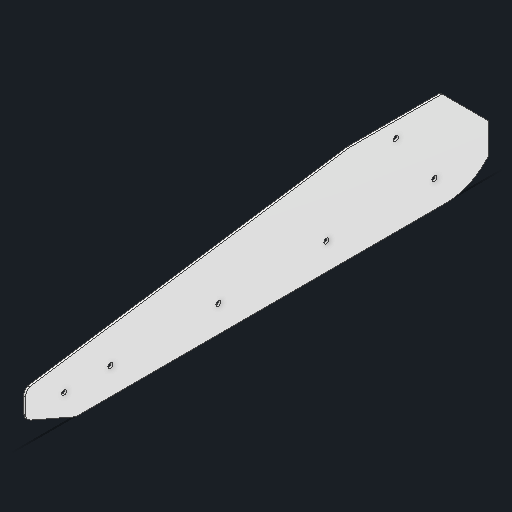
# Autodesk Inventor part: Skirt
Saved by Autodesk Inventor 2025.1 (Build 291241000, 241)
## iProperties
Created: 2024-10-17
Part Number: Skirt
Material: Acetal Resin, White
Document SubType Name: Sheet Metal
Designer: averey
Density: 1.425 g/cm^3
Appearance: Smooth - White
Mass: 37.0306 g
Surface Area: 482.458 cm^2
Volume: 37.0306 cm^3
Flat Pattern Width: 7.9375 cm
Flat Pattern Length: 38.1 cm
Flat Pattern Area: 302.419 cm^2
Sheet Metal Rule: Default_mm
Sheet Metal Width: 3.125 in
Sheet Metal Length: 15.000 in
Sheet Metal Area: 46.875 in^2
d0: 0.500 in
d1: 12.000 in
d2: 0.625 in
d3: 1.000 in
d4: 0.125 in
d8: 0.165 in
Author: averey
Autodesk Inventor part; units mm, degrees
ref_plane "YZ Plane" through (0, 0, 0) normal (1, 0, 0) x (0, 1, 0)
ref_plane "XZ Plane" through (0, 0, 0) normal (0, 1, 0) x (-1, 0, 0)
ref_plane "XY Plane" through (0, 0, 0) normal (0, 0, 1) x (1, 0, 0)
sketch "main" plane through (0, 0, 0) normal (0, 0, 1) x (1, 0, 0)
  circle A0 centre (-12.3674, 169.8166) radius 2.0955
  circle A1 centre (-12.3674, 131.7166) radius 2.0955
  circle A2 centre (-12.3674, 42.8166) radius 2.0955
  circle A3 centre (-12.3674, -46.0834) radius 2.0955
  circle A4 centre (-12.3674, -134.9834) radius 2.0955
  arc A5 (6.5152, 193.7683) -> (0.3326, 201.5666) centre (0.3326, 195.2166) ccw
  line L0 (-34.5924, 159.4847) -> (-34.5924, -144.653)
  line L1 (5.8319, 198.3916) -> (44.7826, -65.1334)
  arc A6 (-34.3276, 160.7541) -> (-34.5924, 159.4847) centre (-31.4174, 159.4847) ccw
  line L2 (-34.3276, 160.7541) -> (-18.1878, 197.7554)
  line L3 (0.3326, 201.5666) -> (-12.3674, 201.5666)
  arc A7 (-12.3674, 201.5666) -> (-18.1878, 197.7554) centre (-12.3674, 195.2166) ccw
  line L4 (44.7826, -65.1334) -> (44.7826, -141.3334)
  arc A8 (-34.5924, -144.653) -> (-18.7174, -179.4334) centre (11.4451, -144.653) ccw
  line L5 (6.6826, -179.4334) -> (-18.7174, -179.4334)
  line L6 (44.7826, -141.3334) -> (6.6826, -179.4334)
  circle A9 centre (32.0826, -103.2334) radius 2.0955
  point P0 (-1.329, 35.5886)
  point P1 (-34.5924, 160.147)
  point P2 (38.4326, -84.1834)
  dimension "d0" = 12.7
  dimension "d1" = 304.8
  dimension "d2" = 15.875
  dimension "d3" = 25.4
  dimension "d4" = 3.175
  dimension "d8" = 4.191
  dimension "d9" = 4.191
  dimension "d10" = 4.191
  dimension "d11" = 4.191
  dimension "d12" = 4.191
  dimension "d13" = 4.191
  measures "d0" diameter of A5
  measures "d1" distance of point (-34.592, 160.147) L0.end
  measures "d2" distance from line of L5.end L0
  measures "d3" distance of L6.end L5.end
  measures "d4" radius of A6
  measures "d8" diameter of A9
  measures "d9" diameter of A3
  measures "d10" diameter of A4
  measures "d11" diameter of A2
  measures "d12" diameter of A1
  measures "d13" diameter of A0
sketch "Sketch1" plane through (0, 0, 0) normal (1, 0, 0) x (0, 1, 0)
  circle A0 centre (0, 0) radius 2.0955
  circle A1 centre (0, -38.1) radius 2.0955
  circle A2 centre (0, -127) radius 2.0955
  circle A3 centre (0, -215.9) radius 2.0955
  circle A4 centre (0, -304.8) radius 2.0955
  arc A5 (18.8826, 23.9517) -> (12.7, 31.75) centre (12.7, 25.4) ccw
  line L0 (-22.225, -10.3319) -> (-22.225, -314.4696)
  line L1 (18.1993, 28.575) -> (57.15, -234.95)
  arc A6 (-21.9602, -9.0625) -> (-22.225, -10.3319) centre (-19.05, -10.3319) ccw
  line L2 (-21.9602, -9.0625) -> (-5.8204, 27.9388)
  line L3 (12.7, 31.75) -> (0, 31.75)
  arc A7 (0, 31.75) -> (-5.8204, 27.9388) centre (0, 25.4) ccw
  line L4 (57.15, -234.95) -> (57.15, -311.15)
  arc A8 (-22.225, -314.4696) -> (-6.35, -349.25) centre (23.8125, -314.4696) ccw
  line L5 (19.05, -349.25) -> (-6.35, -349.25)
  line L6 (57.15, -311.15) -> (19.05, -349.25)
  circle A9 centre (44.45, -273.05) radius 2.0955
  constraints: 1 other
extrude "Extrusion1" add sketch "Sketch1" along normal blind 1.5875 contours L1 L4 L6 L5 A8 L0 A6 L2 A7 L3 A5
equation "\"BendRadius\" = Thickness"
equation "\"BendReliefWidth\" = Thickness"
equation "\"BendReliefDepth\" = 0.5 * Thickness"
equation "\"CornerReliefSize\" = 4 * Thickness"
equation "\"MinimumRemnant\" = 2 * Thickness"
equation "\"TransitionRadius\" = BendRadius"
equation "\"JacobiRadiusSize\" = BendRadius"
equation "\"GapSize\" = Thickness"
equation "\"Thickness\" = 1.5875"
body "Solid1"
